Autodesk Fusion 360 part; units mm, degrees
(part 2 of 3)
  arc A350 (118.6572, -98.4677) -> (119.1572, -98.9677) centre (119.1572, -98.4677) ccw
  arc A351 (132.1572, -98.9677) -> (132.6572, -98.4677) centre (132.1572, -98.4677) ccw
  line L356 (138.2072, -84.9677) -> (151.2072, -84.9677)
  line L357 (138.2072, -98.9677) -> (151.2072, -98.9677)
  line L358 (137.7072, -85.4677) -> (137.7072, -98.4677)
  line L359 (151.7072, -85.4677) -> (151.7072, -98.4677)
  arc A352 (138.2072, -84.9677) -> (137.7072, -85.4677) centre (138.2072, -85.4677) ccw
  arc A353 (151.7072, -85.4677) -> (151.2072, -84.9677) centre (151.2072, -85.4677) ccw
  arc A354 (137.7072, -98.4677) -> (138.2072, -98.9677) centre (138.2072, -98.4677) ccw
  arc A355 (151.2072, -98.9677) -> (151.7072, -98.4677) centre (151.2072, -98.4677) ccw
  line L360 (157.2572, -84.9677) -> (170.2572, -84.9677)
  line L361 (157.2572, -98.9677) -> (170.2572, -98.9677)
  line L362 (156.7572, -85.4677) -> (156.7572, -98.4677)
  line L363 (170.7572, -85.4677) -> (170.7572, -98.4677)
  arc A356 (157.2572, -84.9677) -> (156.7572, -85.4677) centre (157.2572, -85.4677) ccw
  arc A357 (170.7572, -85.4677) -> (170.2572, -84.9677) centre (170.2572, -85.4677) ccw
  arc A358 (156.7572, -98.4677) -> (157.2572, -98.9677) centre (157.2572, -98.4677) ccw
  arc A359 (170.2572, -98.9677) -> (170.7572, -98.4677) centre (170.2572, -98.4677) ccw
  line L364 (176.3072, -84.9677) -> (189.3072, -84.9677)
  line L365 (176.3072, -98.9677) -> (189.3072, -98.9677)
  line L366 (175.8072, -85.4677) -> (175.8072, -98.4677)
  line L367 (189.8072, -85.4677) -> (189.8072, -98.4677)
  arc A360 (176.3072, -84.9677) -> (175.8072, -85.4677) centre (176.3072, -85.4677) ccw
  arc A361 (189.8072, -85.4677) -> (189.3072, -84.9677) centre (189.3072, -85.4677) ccw
  arc A362 (175.8072, -98.4677) -> (176.3072, -98.9677) centre (176.3072, -98.4677) ccw
  arc A363 (189.3072, -98.9677) -> (189.8072, -98.4677) centre (189.3072, -98.4677) ccw
  line L368 (195.3572, -84.9677) -> (208.3572, -84.9677)
  line L369 (195.3572, -98.9677) -> (208.3572, -98.9677)
  line L370 (194.8572, -85.4677) -> (194.8572, -98.4677)
  line L371 (208.8572, -85.4677) -> (208.8572, -98.4677)
  arc A364 (195.3572, -84.9677) -> (194.8572, -85.4677) centre (195.3572, -85.4677) ccw
  arc A365 (208.8572, -85.4677) -> (208.3572, -84.9677) centre (208.3572, -85.4677) ccw
  arc A366 (194.8572, -98.4677) -> (195.3572, -98.9677) centre (195.3572, -98.4677) ccw
  arc A367 (208.3572, -98.9677) -> (208.8572, -98.4677) centre (208.3572, -98.4677) ccw
  dimension "d1" = 25.211
  dimension "d2" = 19.875
  constraint horizontal L1
  constraint vertical L0
  constraint horizontal L3
  constraint vertical L2
  measures "d1" distance of L2 L326
  measures "d2" distance of L3 L325
extrude "Extrude1" add sketch "Sketch1" along normal blind 2.5
sketch "Sketch3" plane through (0, 0, 2.5) normal (0, 0, 1) x (-1, 0, 0)
  arc A0 (-66.7697, 65.9177) -> (-66.2697, 66.4177) centre (-66.7697, 66.4177) ccw
  line L0 (-66.7697, 65.9177) -> (-79.7697, 65.9177)
  arc A1 (-80.2697, 66.4177) -> (-79.7697, 65.9177) centre (-79.7697, 66.4177) ccw
  line L1 (-80.2697, 66.4177) -> (-80.2697, 79.4177)
  arc A2 (-79.7697, 79.9177) -> (-80.2697, 79.4177) centre (-79.7697, 79.4177) ccw
  line L2 (-79.7697, 79.9177) -> (-66.7697, 79.9177)
  arc A3 (-66.2697, 79.4177) -> (-66.7697, 79.9177) centre (-66.7697, 79.4177) ccw
  line L3 (-66.2697, 79.4177) -> (-66.2697, 66.4177)
  arc A4 (-195.3572, 8.7677) -> (-194.8572, 9.2677) centre (-195.3572, 9.2677) ccw
  line L4 (-195.3572, 8.7677) -> (-208.3572, 8.7677)
  arc A5 (-208.8572, 9.2677) -> (-208.3572, 8.7677) centre (-208.3572, 9.2677) ccw
  line L5 (-208.8572, 9.2677) -> (-208.8572, 22.2677)
  arc A6 (-208.3572, 22.7677) -> (-208.8572, 22.2677) centre (-208.3572, 22.2677) ccw
  line L6 (-208.3572, 22.7677) -> (-195.3572, 22.7677)
  arc A7 (-194.8572, 22.2677) -> (-195.3572, 22.7677) centre (-195.3572, 22.2677) ccw
  line L7 (-194.8572, 22.2677) -> (-194.8572, 9.2677)
  arc A8 (-14.3822, 27.8177) -> (-13.8822, 28.3177) centre (-14.3822, 28.3177) ccw
  line L8 (-14.3822, 27.8177) -> (-27.3822, 27.8177)
  arc A9 (-27.8822, 28.3177) -> (-27.3822, 27.8177) centre (-27.3822, 28.3177) ccw
  line L9 (-27.8822, 28.3177) -> (-27.8822, 41.3177)
  arc A10 (-27.3822, 41.8177) -> (-27.8822, 41.3177) centre (-27.3822, 41.3177) ccw
  line L10 (-27.3822, 41.8177) -> (-14.3822, 41.8177)
  arc A11 (-13.8822, 41.3177) -> (-14.3822, 41.8177) centre (-14.3822, 41.3177) ccw
  line L11 (-13.8822, 41.3177) -> (-13.8822, 28.3177)
  arc A12 (85.6303, 27.8177) -> (86.1303, 28.3177) centre (85.6303, 28.3177) ccw
  line L12 (85.6303, 27.8177) -> (72.6303, 27.8177)
  arc A13 (72.1303, 28.3177) -> (72.6303, 27.8177) centre (72.6303, 28.3177) ccw
  line L13 (72.1303, 28.3177) -> (72.1303, 41.3177)
  arc A14 (72.6303, 41.8177) -> (72.1303, 41.3177) centre (72.6303, 41.3177) ccw
  line L14 (72.6303, 41.8177) -> (85.6303, 41.8177)
  arc A15 (86.1303, 41.3177) -> (85.6303, 41.8177) centre (85.6303, 41.3177) ccw
  line L15 (86.1303, 41.3177) -> (86.1303, 28.3177)
  arc A16 (-119.1572, -10.2823) -> (-118.6572, -9.7823) centre (-119.1572, -9.7823) ccw
  line L16 (-119.1572, -10.2823) -> (-132.1572, -10.2823)
  arc A17 (-132.6572, -9.7823) -> (-132.1572, -10.2823) centre (-132.1572, -9.7823) ccw
  line L17 (-132.6572, -9.7823) -> (-132.6572, 3.2177)
  arc A18 (-132.1572, 3.7177) -> (-132.6572, 3.2177) centre (-132.1572, 3.2177) ccw
  line L18 (-132.1572, 3.7177) -> (-119.1572, 3.7177)
  arc A19 (-118.6572, 3.2177) -> (-119.1572, 3.7177) centre (-119.1572, 3.2177) ccw
  line L19 (-118.6572, 3.2177) -> (-118.6572, -9.7823)
  arc A20 (-4.8572, -10.2823) -> (-4.3572, -9.7823) centre (-4.8572, -9.7823) ccw
  line L20 (-4.8572, -10.2823) -> (-17.8572, -10.2823)
  arc A21 (-18.3572, -9.7823) -> (-17.8572, -10.2823) centre (-17.8572, -9.7823) ccw
  line L21 (-18.3572, -9.7823) -> (-18.3572, 3.2177)
  arc A22 (-17.8572, 3.7177) -> (-18.3572, 3.2177) centre (-17.8572, 3.2177) ccw
  line L22 (-17.8572, 3.7177) -> (-4.8572, 3.7177)
  arc A23 (-4.3572, 3.2177) -> (-4.8572, 3.7177) centre (-4.8572, 3.2177) ccw
  line L23 (-4.3572, 3.2177) -> (-4.3572, -9.7823)
  arc A24 (-104.8697, 65.9177) -> (-104.3697, 66.4177) centre (-104.8697, 66.4177) ccw
  line L24 (-104.8697, 65.9177) -> (-117.8697, 65.9177)
  arc A25 (-118.3697, 66.4177) -> (-117.8697, 65.9177) centre (-117.8697, 66.4177) ccw
  line L25 (-118.3697, 66.4177) -> (-118.3697, 79.4177)
  arc A26 (-117.8697, 79.9177) -> (-118.3697, 79.4177) centre (-117.8697, 79.4177) ccw
  line L26 (-117.8697, 79.9177) -> (-104.8697, 79.9177)
  arc A27 (-104.3697, 79.4177) -> (-104.8697, 79.9177) centre (-104.8697, 79.4177) ccw
  line L27 (-104.3697, 79.4177) -> (-104.3697, 66.4177)
  arc A28 (-23.9072, -10.2823) -> (-23.4072, -9.7823) centre (-23.9072, -9.7823) ccw
  line L28 (-23.9072, -10.2823) -> (-36.9072, -10.2823)
  arc A29 (-37.4072, -9.7823) -> (-36.9072, -10.2823) centre (-36.9072, -9.7823) ccw
  line L29 (-37.4072, -9.7823) -> (-37.4072, 3.2177)
  arc A30 (-36.9072, 3.7177) -> (-37.4072, 3.2177) centre (-36.9072, 3.2177) ccw
  line L30 (-36.9072, 3.7177) -> (-23.9072, 3.7177)
  arc A31 (-23.4072, 3.2177) -> (-23.9072, 3.7177) centre (-23.9072, 3.2177) ccw
  line L31 (-23.4072, 3.2177) -> (-23.4072, -9.7823)
  arc A32 (52.2928, 8.7677) -> (52.7928, 9.2677) centre (52.2928, 9.2677) ccw
  line L32 (52.2928, 8.7677) -> (39.2928, 8.7677)
  arc A33 (38.7928, 9.2677) -> (39.2928, 8.7677) centre (39.2928, 9.2677) ccw
  line L33 (38.7928, 9.2677) -> (38.7928, 22.2677)
  arc A34 (39.2928, 22.7677) -> (38.7928, 22.2677) centre (39.2928, 22.2677) ccw
  line L34 (39.2928, 22.7677) -> (52.2928, 22.7677)
  arc A35 (52.7928, 22.2677) -> (52.2928, 22.7677) centre (52.2928, 22.2677) ccw
  line L35 (52.7928, 22.2677) -> (52.7928, 9.2677)
  arc A36 (86.9246, 66.9177) -> (87.4246, 67.4177) centre (86.9246, 67.4177) ccw
  line L36 (86.9246, 66.9177) -> (80.9246, 66.9177)
  arc A37 (80.4246, 67.4177) -> (80.9246, 66.9177) centre (80.9246, 67.4177) ccw
  line L37 (80.4246, 67.4177) -> (80.4246, 81.4177)
  arc A38 (80.9246, 81.9177) -> (80.4246, 81.4177) centre (80.9246, 81.4177) ccw
  line L38 (80.9246, 81.9177) -> (86.9246, 81.9177)
  arc A39 (87.4246, 81.4177) -> (86.9246, 81.9177) centre (86.9246, 81.4177) ccw
  line L39 (87.4246, 81.4177) -> (87.4246, 67.4177)
  arc A40 (-155.9629, 47.8677) -> (-155.4629, 48.3677) centre (-155.9629, 48.3677) ccw
  line L40 (-155.9629, 47.8677) -> (-161.9629, 47.8677)
  arc A41 (-162.4629, 48.3677) -> (-161.9629, 47.8677) centre (-161.9629, 48.3677) ccw
  line L41 (-162.4629, 48.3677) -> (-162.4629, 62.3677)
  arc A42 (-161.9629, 62.8677) -> (-162.4629, 62.3677) centre (-161.9629, 62.3677) ccw
  line L42 (-161.9629, 62.8677) -> (-155.9629, 62.8677)
  arc A43 (-155.4629, 62.3677) -> (-155.9629, 62.8677) centre (-155.9629, 62.3677) ccw
  line L43 (-155.4629, 62.3677) -> (-155.4629, 48.3677)
  arc A44 (-23.9072, 8.7677) -> (-23.4072, 9.2677) centre (-23.9072, 9.2677) ccw
  line L44 (-23.9072, 8.7677) -> (-36.9072, 8.7677)
  arc A45 (-37.4072, 9.2677) -> (-36.9072, 8.7677) centre (-36.9072, 9.2677) ccw
  line L45 (-37.4072, 9.2677) -> (-37.4072, 22.2677)
  arc A46 (-36.9072, 22.7677) -> (-37.4072, 22.2677) centre (-36.9072, 22.2677) ccw
  line L46 (-36.9072, 22.7677) -> (-23.9072, 22.7677)
  arc A47 (-23.4072, 22.2677) -> (-23.9072, 22.7677) centre (-23.9072, 22.2677) ccw
  line L47 (-23.4072, 22.2677) -> (-23.4072, 9.2677)
  arc A48 (88.0116, 84.9677) -> (88.5116, 85.4677) centre (88.0116, 85.4677) ccw
  line L48 (88.0116, 84.9677) -> (75.0116, 84.9677)
  arc A49 (74.5116, 85.4677) -> (75.0116, 84.9677) centre (75.0116, 85.4677) ccw
  line L49 (74.5116, 85.4677) -> (74.5116, 98.4677)
  arc A50 (75.0116, 98.9677) -> (74.5116, 98.4677) centre (75.0116, 98.4677) ccw
  line L50 (75.0116, 98.9677) -> (88.0116, 98.9677)
  arc A51 (88.5116, 98.4677) -> (88.0116, 98.9677) centre (88.0116, 98.4677) ccw
  line L51 (88.5116, 98.4677) -> (88.5116, 85.4677)
  arc A52 (-133.4447, 46.8677) -> (-132.9447, 47.3677) centre (-133.4447, 47.3677) ccw
  line L52 (-133.4447, 46.8677) -> (-146.4447, 46.8677)
  arc A53 (-146.9447, 47.3677) -> (-146.4447, 46.8677) centre (-146.4447, 47.3677) ccw
  line L53 (-146.9447, 47.3677) -> (-146.9447, 60.3677)
  arc A54 (-146.4447, 60.8677) -> (-146.9447, 60.3677) centre (-146.4447, 60.3677) ccw
  line L54 (-146.4447, 60.8677) -> (-133.4447, 60.8677)
  arc A55 (-132.9447, 60.3677) -> (-133.4447, 60.8677) centre (-133.4447, 60.3677) ccw
  line L55 (-132.9447, 60.3677) -> (-132.9447, 47.3677)
  arc A56 (-171.5447, 27.8177) -> (-171.0447, 28.3177) centre (-171.5447, 28.3177) ccw
  line L56 (-171.5447, 27.8177) -> (-184.5447, 27.8177)
  arc A57 (-185.0447, 28.3177) -> (-184.5447, 27.8177) centre (-184.5447, 28.3177) ccw
  line L57 (-185.0447, 28.3177) -> (-185.0447, 41.3177)
  arc A58 (-184.5447, 41.8177) -> (-185.0447, 41.3177) centre (-184.5447, 41.3177) ccw
  line L58 (-184.5447, 41.8177) -> (-171.5447, 41.8177)
  arc A59 (-171.0447, 41.3177) -> (-171.5447, 41.8177) centre (-171.5447, 41.3177) ccw
  line L59 (-171.0447, 41.3177) -> (-171.0447, 28.3177)
  arc A60 (-138.2072, -10.2823) -> (-137.7072, -9.7823) centre (-138.2072, -9.7823) ccw
  line L60 (-138.2072, -10.2823) -> (-151.2072, -10.2823)
  arc A61 (-151.7072, -9.7823) -> (-151.2072, -10.2823) centre (-151.2072, -9.7823) ccw
  line L61 (-151.7072, -9.7823) -> (-151.7072, 3.2177)
  arc A62 (-151.2072, 3.7177) -> (-151.7072, 3.2177) centre (-151.2072, 3.2177) ccw
  line L62 (-151.2072, 3.7177) -> (-138.2072, 3.7177)
  arc A63 (-137.7072, 3.2177) -> (-138.2072, 3.7177) centre (-138.2072, 3.2177) ccw
  line L63 (-137.7072, 3.2177) -> (-137.7072, -9.7823)
  arc A64 (-176.3072, -10.2823) -> (-175.8072, -9.7823) centre (-176.3072, -9.7823) ccw
  line L64 (-176.3072, -10.2823) -> (-189.3072, -10.2823)
  arc A65 (-189.8072, -9.7823) -> (-189.3072, -10.2823) centre (-189.3072, -9.7823) ccw
  line L65 (-189.8072, -9.7823) -> (-189.8072, 3.2177)
  arc A66 (-189.3072, 3.7177) -> (-189.8072, 3.2177) centre (-189.3072, 3.2177) ccw
  line L66 (-189.3072, 3.7177) -> (-176.3072, 3.7177)
  arc A67 (-175.8072, 3.2177) -> (-176.3072, 3.7177) centre (-176.3072, 3.2177) ccw
  line L67 (-175.8072, 3.2177) -> (-175.8072, -9.7823)
  arc A68 (4.6678, 27.8177) -> (5.1678, 28.3177) centre (4.6678, 28.3177) ccw
  line L68 (4.6678, 27.8177) -> (-8.3322, 27.8177)
  arc A69 (-8.8322, 28.3177) -> (-8.3322, 27.8177) centre (-8.3322, 28.3177) ccw
  line L69 (-8.8322, 28.3177) -> (-8.8322, 41.3177)
  arc A70 (-8.3322, 41.8177) -> (-8.8322, 41.3177) centre (-8.3322, 41.3177) ccw
  line L70 (-8.3322, 41.8177) -> (4.6678, 41.8177)
  arc A71 (5.1678, 41.3177) -> (4.6678, 41.8177) centre (4.6678, 41.3177) ccw
  line L71 (5.1678, 41.3177) -> (5.1678, 28.3177)
  arc A72 (64.1991, 84.9677) -> (64.6991, 85.4677) centre (64.1991, 85.4677) ccw
  line L72 (64.1991, 84.9677) -> (51.1991, 84.9677)
  arc A73 (50.6991, 85.4677) -> (51.1991, 84.9677) centre (51.1991, 85.4677) ccw
  line L73 (50.6991, 85.4677) -> (50.6991, 98.4677)
  arc A74 (51.1991, 98.9677) -> (50.6991, 98.4677) centre (51.1991, 98.4677) ccw
  line L74 (51.1991, 98.9677) -> (64.1991, 98.9677)
  arc A75 (64.6991, 98.4677) -> (64.1991, 98.9677) centre (64.1991, 98.4677) ccw
  line L75 (64.6991, 98.4677) -> (64.6991, 85.4677)
  arc A76 (52.2928, -10.2823) -> (52.7928, -9.7823) centre (52.2928, -9.7823) ccw
  line L76 (52.2928, -10.2823) -> (39.2928, -10.2823)
  arc A77 (38.7928, -9.7823) -> (39.2928, -10.2823) centre (39.2928, -9.7823) ccw
  line L77 (38.7928, -9.7823) -> (38.7928, 3.2177)
  arc A78 (39.2928, 3.7177) -> (38.7928, 3.2177) centre (39.2928, 3.2177) ccw
  line L78 (39.2928, 3.7177) -> (52.2928, 3.7177)
  arc A79 (52.7928, 3.2177) -> (52.2928, 3.7177) centre (52.2928, 3.2177) ccw
  line L79 (52.7928, 3.2177) -> (52.7928, -9.7823)
  arc A80 (-109.6322, 27.8177) -> (-109.1322, 28.3177) centre (-109.6322, 28.3177) ccw
  line L80 (-109.6322, 27.8177) -> (-122.6322, 27.8177)
  arc A81 (-123.1322, 28.3177) -> (-122.6322, 27.8177) centre (-122.6322, 28.3177) ccw
  line L81 (-123.1322, 28.3177) -> (-123.1322, 41.3177)
  arc A82 (-122.6322, 41.8177) -> (-123.1322, 41.3177) centre (-122.6322, 41.3177) ccw
  line L82 (-122.6322, 41.8177) -> (-109.6322, 41.8177)
  arc A83 (-109.1322, 41.3177) -> (-109.6322, 41.8177) centre (-109.6322, 41.3177) ccw
  line L83 (-109.1322, 41.3177) -> (-109.1322, 28.3177)
  arc A84 (42.7678, 27.8177) -> (43.2678, 28.3177) centre (42.7678, 28.3177) ccw
  line L84 (42.7678, 27.8177) -> (29.7678, 27.8177)
  arc A85 (29.2678, 28.3177) -> (29.7678, 27.8177) centre (29.7678, 28.3177) ccw
  line L85 (29.2678, 28.3177) -> (29.2678, 41.3177)
  arc A86 (29.7678, 41.8177) -> (29.2678, 41.3177) centre (29.7678, 41.3177) ccw
  line L86 (29.7678, 41.8177) -> (42.7678, 41.8177)
  arc A87 (43.2678, 41.3177) -> (42.7678, 41.8177) centre (42.7678, 41.3177) ccw
  line L87 (43.2678, 41.3177) -> (43.2678, 28.3177)
  arc A88 (-100.1072, 8.7677) -> (-99.6072, 9.2677) centre (-100.1072, 9.2677) ccw
  line L88 (-100.1072, 8.7677) -> (-113.1072, 8.7677)
  arc A89 (-113.6072, 9.2677) -> (-113.1072, 8.7677) centre (-113.1072, 9.2677) ccw
  line L89 (-113.6072, 9.2677) -> (-113.6072, 22.2677)
  arc A90 (-113.1072, 22.7677) -> (-113.6072, 22.2677) centre (-113.1072, 22.2677) ccw
  line L90 (-113.1072, 22.7677) -> (-100.1072, 22.7677)
  arc A91 (-99.6072, 22.2677) -> (-100.1072, 22.7677) centre (-100.1072, 22.2677) ccw
  line L91 (-99.6072, 22.2677) -> (-99.6072, 9.2677)
  arc A92 (-0.0947, 46.8677) -> (0.4053, 47.3677) centre (-0.0947, 47.3677) ccw
  line L92 (-0.0947, 46.8677) -> (-13.0947, 46.8677)
  arc A93 (-13.5947, 47.3677) -> (-13.0947, 46.8677) centre (-13.0947, 47.3677) ccw
  line L93 (-13.5947, 47.3677) -> (-13.5947, 60.3677)
  arc A94 (-13.0947, 60.8677) -> (-13.5947, 60.3677) centre (-13.0947, 60.3677) ccw
  line L94 (-13.0947, 60.8677) -> (-0.0947, 60.8677)
  arc A95 (0.4053, 60.3677) -> (-0.0947, 60.8677) centre (-0.0947, 60.3677) ccw
  line L95 (0.4053, 60.3677) -> (0.4053, 47.3677)
  arc A96 (63.0486, 66.9177) -> (63.5486, 67.4177) centre (63.0486, 67.4177) ccw
  line L96 (63.0486, 66.9177) -> (57.0486, 66.9177)
  arc A97 (56.5486, 67.4177) -> (57.0486, 66.9177) centre (57.0486, 67.4177) ccw
  line L97 (56.5486, 67.4177) -> (56.5486, 81.4177)
  arc A98 (57.0486, 81.9177) -> (56.5486, 81.4177) centre (57.0486, 81.4177) ccw
  line L98 (57.0486, 81.9177) -> (63.0486, 81.9177)
  arc A99 (63.5486, 81.4177) -> (63.0486, 81.9177) centre (63.0486, 81.4177) ccw
  line L99 (63.5486, 81.4177) -> (63.5486, 67.4177)
  arc A100 (-33.4322, 27.8177) -> (-32.9322, 28.3177) centre (-33.4322, 28.3177) ccw
  line L100 (-33.4322, 27.8177) -> (-46.4322, 27.8177)
  arc A101 (-46.9322, 28.3177) -> (-46.4322, 27.8177) centre (-46.4322, 28.3177) ccw
  line L101 (-46.9322, 28.3177) -> (-46.9322, 41.3177)
  arc A102 (-46.4322, 41.8177) -> (-46.9322, 41.3177) centre (-46.4322, 41.3177) ccw
  line L102 (-46.4322, 41.8177) -> (-33.4322, 41.8177)
  arc A103 (-32.9322, 41.3177) -> (-33.4322, 41.8177) centre (-33.4322, 41.3177) ccw
  line L103 (-32.9322, 41.3177) -> (-32.9322, 28.3177)
  arc A104 (-195.3572, 27.8177) -> (-194.8572, 28.3177) centre (-195.3572, 28.3177) ccw
  line L104 (-195.3572, 27.8177) -> (-208.3572, 27.8177)
  arc A105 (-208.8572, 28.3177) -> (-208.3572, 27.8177) centre (-208.3572, 28.3177) ccw
  line L105 (-208.8572, 28.3177) -> (-208.8572, 41.3177)
  arc A106 (-208.3572, 41.8177) -> (-208.8572, 41.3177) centre (-208.3572, 41.3177) ccw
  line L106 (-208.3572, 41.8177) -> (-195.3572, 41.8177)
  arc A107 (-194.8572, 41.3177) -> (-195.3572, 41.8177) centre (-195.3572, 41.3177) ccw
  line L107 (-194.8572, 41.3177) -> (-194.8572, 28.3177)
  arc A108 (-176.3072, 65.9177) -> (-175.8072, 66.4177) centre (-176.3072, 66.4177) ccw
  line L108 (-176.3072, 65.9177) -> (-189.3072, 65.9177)
  arc A109 (-189.8072, 66.4177) -> (-189.3072, 65.9177) centre (-189.3072, 66.4177) ccw
  line L109 (-189.8072, 66.4177) -> (-189.8072, 79.4177)
  arc A110 (-189.3072, 79.9177) -> (-189.8072, 79.4177) centre (-189.3072, 79.4177) ccw
  line L110 (-189.3072, 79.9177) -> (-176.3072, 79.9177)
  arc A111 (-175.8072, 79.4177) -> (-176.3072, 79.9177) centre (-176.3072, 79.4177) ccw
  line L111 (-175.8072, 79.4177) -> (-175.8072, 66.4177)
  arc A112 (-100.1072, -10.2823) -> (-99.6072, -9.7823) centre (-100.1072, -9.7823) ccw
  line L112 (-100.1072, -10.2823) -> (-113.1072, -10.2823)
  arc A113 (-113.6072, -9.7823) -> (-113.1072, -10.2823) centre (-113.1072, -9.7823) ccw
  line L113 (-113.6072, -9.7823) -> (-113.6072, 3.2177)
  arc A114 (-113.1072, 3.7177) -> (-113.6072, 3.2177) centre (-113.1072, 3.2177) ccw
  line L114 (-113.1072, 3.7177) -> (-100.1072, 3.7177)
  arc A115 (-99.6072, 3.2177) -> (-100.1072, 3.7177) centre (-100.1072, 3.2177) ccw
  line L115 (-99.6072, 3.2177) -> (-99.6072, -9.7823)
  arc A116 (-157.2572, -10.2823) -> (-156.7572, -9.7823) centre (-157.2572, -9.7823) ccw
  line L116 (-157.2572, -10.2823) -> (-170.2572, -10.2823)
  arc A117 (-170.7572, -9.7823) -> (-170.2572, -10.2823) centre (-170.2572, -9.7823) ccw
  line L117 (-170.7572, -9.7823) -> (-170.7572, 3.2177)
  arc A118 (-170.2572, 3.7177) -> (-170.7572, 3.2177) centre (-170.2572, 3.2177) ccw
  line L118 (-170.2572, 3.7177) -> (-157.2572, 3.7177)
  arc A119 (-156.7572, 3.2177) -> (-157.2572, 3.7177) centre (-157.2572, 3.2177) ccw
  line L119 (-156.7572, 3.2177) -> (-156.7572, -9.7823)
  arc A120 (33.2428, 8.7677) -> (33.7428, 9.2677) centre (33.2428, 9.2677) ccw
  line L120 (33.2428, 8.7677) -> (20.2428, 8.7677)
  arc A121 (19.7428, 9.2677) -> (20.2428, 8.7677) centre (20.2428, 9.2677) ccw
  line L121 (19.7428, 9.2677) -> (19.7428, 22.2677)
  arc A122 (20.2428, 22.7677) -> (19.7428, 22.2677) centre (20.2428, 22.2677) ccw
  line L122 (20.2428, 22.7677) -> (33.2428, 22.7677)
  arc A123 (33.7428, 22.2677) -> (33.2428, 22.7677) centre (33.2428, 22.2677) ccw
  line L123 (33.7428, 22.2677) -> (33.7428, 9.2677)
  arc A124 (90.3928, -10.2823) -> (90.8928, -9.7823) centre (90.3928, -9.7823) ccw
  line L124 (90.3928, -10.2823) -> (77.3928, -10.2823)
  arc A125 (76.8928, -9.7823) -> (77.3928, -10.2823) centre (77.3928, -9.7823) ccw
  line L125 (76.8928, -9.7823) -> (76.8928, 3.2177)
  arc A126 (77.3928, 3.7177) -> (76.8928, 3.2177) centre (77.3928, 3.2177) ccw
  line L126 (77.3928, 3.7177) -> (90.3928, 3.7177)
  arc A127 (90.8928, 3.2177) -> (90.3928, 3.7177) centre (90.3928, 3.2177) ccw
  line L127 (90.8928, 3.2177) -> (90.8928, -9.7823)
  arc A128 (18.9553, 46.8677) -> (19.4553, 47.3677) centre (18.9553, 47.3677) ccw
  line L128 (18.9553, 46.8677) -> (5.9553, 46.8677)
  arc A129 (5.4553, 47.3677) -> (5.9553, 46.8677) centre (5.9553, 47.3677) ccw
  line L129 (5.4553, 47.3677) -> (5.4553, 60.3677)
  arc A130 (5.9553, 60.8677) -> (5.4553, 60.3677) centre (5.9553, 60.3677) ccw
  line L130 (5.9553, 60.8677) -> (18.9553, 60.8677)
  arc A131 (19.4553, 60.3677) -> (18.9553, 60.8677) centre (18.9553, 60.3677) ccw
  line L131 (19.4553, 60.3677) -> (19.4553, 47.3677)
  arc A132 (-71.5322, 27.8177) -> (-71.0322, 28.3177) centre (-71.5322, 28.3177) ccw
  line L132 (-71.5322, 27.8177) -> (-84.5322, 27.8177)
  arc A133 (-85.0322, 28.3177) -> (-84.5322, 27.8177) centre (-84.5322, 28.3177) ccw
  line L133 (-85.0322, 28.3177) -> (-85.0322, 41.3177)
  arc A134 (-84.5322, 41.8177) -> (-85.0322, 41.3177) centre (-84.5322, 41.3177) ccw
  line L134 (-84.5322, 41.8177) -> (-71.5322, 41.8177)
  arc A135 (-71.0322, 41.3177) -> (-71.5322, 41.8177) centre (-71.5322, 41.3177) ccw
  line L135 (-71.0322, 41.3177) -> (-71.0322, 28.3177)
  arc A136 (-114.3947, 46.8677) -> (-113.8947, 47.3677) centre (-114.3947, 47.3677) ccw
  line L136 (-114.3947, 46.8677) -> (-127.3947, 46.8677)
  arc A137 (-127.8947, 47.3677) -> (-127.3947, 46.8677) centre (-127.3947, 47.3677) ccw
  line L137 (-127.8947, 47.3677) -> (-127.8947, 60.3677)
  arc A138 (-127.3947, 60.8677) -> (-127.8947, 60.3677) centre (-127.3947, 60.3677) ccw
  line L138 (-127.3947, 60.8677) -> (-114.3947, 60.8677)
  arc A139 (-113.8947, 60.3677) -> (-114.3947, 60.8677) centre (-114.3947, 60.3677) ccw
  line L139 (-113.8947, 60.3677) -> (-113.8947, 47.3677)
  arc A140 (-81.0572, -10.2823) -> (-80.5572, -9.7823) centre (-81.0572, -9.7823) ccw
  line L140 (-81.0572, -10.2823) -> (-94.0572, -10.2823)
  arc A141 (-94.5572, -9.7823) -> (-94.0572, -10.2823) centre (-94.0572, -9.7823) ccw
  line L141 (-94.5572, -9.7823) -> (-94.5572, 3.2177)
  arc A142 (-94.0572, 3.7177) -> (-94.5572, 3.2177) centre (-94.0572, 3.2177) ccw
  line L142 (-94.0572, 3.7177) -> (-81.0572, 3.7177)
  arc A143 (-80.5572, 3.2177) -> (-81.0572, 3.7177) centre (-81.0572, 3.2177) ccw
  line L143 (-80.5572, 3.2177) -> (-80.5572, -9.7823)
  arc A144 (15.4491, 85.9677) -> (15.9491, 86.4677) centre (15.4491, 86.4677) ccw
  line L144 (15.4491, 85.9677) -> (9.4491, 85.9677)
  arc A145 (8.9491, 86.4677) -> (9.4491, 85.9677) centre (9.4491, 86.4677) ccw
  line L145 (8.9491, 86.4677) -> (8.9491, 100.4677)
  arc A146 (9.4491, 100.9677) -> (8.9491, 100.4677) centre (9.4491, 100.4677) ccw
  line L146 (9.4491, 100.9677) -> (15.4491, 100.9677)
  arc A147 (15.9491, 100.4677) -> (15.4491, 100.9677) centre (15.4491, 100.4677) ccw
  line L147 (15.9491, 100.4677) -> (15.9491, 86.4677)
  arc A148 (-195.3572, 84.9677) -> (-194.8572, 85.4677) centre (-195.3572, 85.4677) ccw
  line L148 (-195.3572, 84.9677) -> (-208.3572, 84.9677)
  arc A149 (-208.8572, 85.4677) -> (-208.3572, 84.9677) centre (-208.3572, 85.4677) ccw
  line L149 (-208.8572, 85.4677) -> (-208.8572, 98.4677)
  arc A150 (-208.3572, 98.9677) -> (-208.8572, 98.4677) centre (-208.3572, 98.4677) ccw
  line L150 (-208.3572, 98.9677) -> (-195.3572, 98.9677)
  arc A151 (-194.8572, 98.4677) -> (-195.3572, 98.9677) centre (-195.3572, 98.4677) ccw
  line L151 (-194.8572, 98.4677) -> (-194.8572, 85.4677)
  arc A152 (-138.2072, 84.9677) -> (-137.7072, 85.4677) centre (-138.2072, 85.4677) ccw
  line L152 (-138.2072, 84.9677) -> (-151.2072, 84.9677)
  arc A153 (-151.7072, 85.4677) -> (-151.2072, 84.9677) centre (-151.2072, 85.4677) ccw
  line L153 (-151.7072, 85.4677) -> (-151.7072, 98.4677)
  arc A154 (-151.2072, 98.9677) -> (-151.7072, 98.4677) centre (-151.2072, 98.4677) ccw
  line L154 (-151.2072, 98.9677) -> (-138.2072, 98.9677)
  arc A155 (-137.7072, 98.4677) -> (-138.2072, 98.9677) centre (-138.2072, 98.4677) ccw
  line L155 (-137.7072, 98.4677) -> (-137.7072, 85.4677)
  arc A156 (83.2491, 46.8677) -> (83.7491, 47.3677) centre (83.2491, 47.3677) ccw
  line L156 (83.2491, 46.8677) -> (70.2491, 46.8677)
  arc A157 (69.7491, 47.3677) -> (70.2491, 46.8677) centre (70.2491, 47.3677) ccw
  line L157 (69.7491, 47.3677) -> (69.7491, 60.3677)
  arc A158 (70.2491, 60.8677) -> (69.7491, 60.3677) centre (70.2491, 60.3677) ccw
  line L158 (70.2491, 60.8677) -> (83.2491, 60.8677)
  arc A159 (83.7491, 60.3677) -> (83.2491, 60.8677) centre (83.2491, 60.3677) ccw
  line L159 (83.7491, 60.3677) -> (83.7491, 47.3677)
  arc A160 (-166.7822, 8.7677) -> (-166.2822, 9.2677) centre (-166.7822, 9.2677) ccw
  line L160 (-166.7822, 8.7677) -> (-179.7822, 8.7677)
  arc A161 (-180.2822, 9.2677) -> (-179.7822, 8.7677) centre (-179.7822, 9.2677) ccw
  line L161 (-180.2822, 9.2677) -> (-180.2822, 22.2677)
  arc A162 (-179.7822, 22.7677) -> (-180.2822, 22.2677) centre (-179.7822, 22.2677) ccw
  line L162 (-179.7822, 22.7677) -> (-166.7822, 22.7677)
  arc A163 (-166.2822, 22.2677) -> (-166.7822, 22.7677) centre (-166.7822, 22.2677) ccw
  line L163 (-166.2822, 22.2677) -> (-166.2822, 9.2677)
  arc A164 (-195.3572, 46.8677) -> (-194.8572, 47.3677) centre (-195.3572, 47.3677) ccw
  line L164 (-195.3572, 46.8677) -> (-208.3572, 46.8677)
  arc A165 (-208.8572, 47.3677) -> (-208.3572, 46.8677) centre (-208.3572, 47.3677) ccw
  line L165 (-208.8572, 47.3677) -> (-208.8572, 60.3677)
  arc A166 (-208.3572, 60.8677) -> (-208.8572, 60.3677) centre (-208.3572, 60.3677) ccw
  line L166 (-208.3572, 60.8677) -> (-195.3572, 60.8677)
  arc A167 (-194.8572, 60.3677) -> (-195.3572, 60.8677) centre (-195.3572, 60.3677) ccw
  line L167 (-194.8572, 60.3677) -> (-194.8572, 47.3677)
  line L168 (-228.9474, 118.8427) -> (-228.9474, -57.4273)
  line L169 (-228.9474, -57.4273) -> (113.7226, -57.4273)
  line L170 (113.7226, -57.4273) -> (113.7226, 118.8427)
  line L171 (113.7226, 118.8427) -> (-228.9474, 118.8427)
  arc A168 (-182.2202, 9.7677) -> (-181.7202, 10.2677) centre (-182.2202, 10.2677) ccw
  line L172 (-182.2202, 9.7677) -> (-188.2202, 9.7677)
  arc A169 (-188.7202, 10.2677) -> (-188.2202, 9.7677) centre (-188.2202, 10.2677) ccw
  line L173 (-188.7202, 10.2677) -> (-188.7202, 24.2677)
  arc A170 (-188.2202, 24.7677) -> (-188.7202, 24.2677) centre (-188.2202, 24.2677) ccw
  line L174 (-188.2202, 24.7677) -> (-182.2202, 24.7677)
  arc A171 (-181.7202, 24.2677) -> (-182.2202, 24.7677) centre (-182.2202, 24.2677) ccw
  line L175 (-181.7202, 24.2677) -> (-181.7202, 10.2677)
  arc A172 (-76.2947, 46.8677) -> (-75.7947, 47.3677) centre (-76.2947, 47.3677) ccw
  line L176 (-76.2947, 46.8677) -> (-89.2947, 46.8677)
  arc A173 (-89.7947, 47.3677) -> (-89.2947, 46.8677) centre (-89.2947, 47.3677) ccw
  line L177 (-89.7947, 47.3677) -> (-89.7947, 60.3677)
  arc A174 (-89.2947, 60.8677) -> (-89.7947, 60.3677) centre (-89.2947, 60.3677) ccw
  line L178 (-89.2947, 60.8677) -> (-76.2947, 60.8677)
  arc A175 (-75.7947, 60.3677) -> (-76.2947, 60.8677) centre (-76.2947, 60.3677) ccw
  line L179 (-75.7947, 60.3677) -> (-75.7947, 47.3677)
  arc A176 (-138.2072, 8.7677) -> (-137.7072, 9.2677) centre (-138.2072, 9.2677) ccw
  line L180 (-138.2072, 8.7677) -> (-151.2072, 8.7677)
  arc A177 (-151.7072, 9.2677) -> (-151.2072, 8.7677) centre (-151.2072, 9.2677) ccw
  line L181 (-151.7072, 9.2677) -> (-151.7072, 22.2677)
  arc A178 (-151.2072, 22.7677) -> (-151.7072, 22.2677) centre (-151.2072, 22.2677) ccw
  line L182 (-151.2072, 22.7677) -> (-138.2072, 22.7677)
  arc A179 (-137.7072, 22.2677) -> (-138.2072, 22.7677) centre (-138.2072, 22.2677) ccw
  line L183 (-137.7072, 22.2677) -> (-137.7072, 9.2677)
  arc A180 (-164.4009, 46.8677) -> (-163.9009, 47.3677) centre (-164.4009, 47.3677) ccw
  line L184 (-164.4009, 46.8677) -> (-177.4009, 46.8677)
  arc A181 (-177.9009, 47.3677) -> (-177.4009, 46.8677) centre (-177.4009, 47.3677) ccw
  line L185 (-177.9009, 47.3677) -> (-177.9009, 60.3677)
  arc A182 (-177.4009, 60.8677) -> (-177.9009, 60.3677) centre (-177.4009, 60.3677) ccw
  line L186 (-177.4009, 60.8677) -> (-164.4009, 60.8677)
  arc A183 (-163.9009, 60.3677) -> (-164.4009, 60.8677) centre (-164.4009, 60.3677) ccw
  line L187 (-163.9009, 60.3677) -> (-163.9009, 47.3677)
  arc A184 (-42.9572, 8.7677) -> (-42.4572, 9.2677) centre (-42.9572, 9.2677) ccw
  line L188 (-42.9572, 8.7677) -> (-55.9572, 8.7677)
  arc A185 (-56.4572, 9.2677) -> (-55.9572, 8.7677) centre (-55.9572, 9.2677) ccw
  line L189 (-56.4572, 9.2677) -> (-56.4572, 22.2677)
  arc A186 (-55.9572, 22.7677) -> (-56.4572, 22.2677) centre (-55.9572, 22.2677) ccw
  line L190 (-55.9572, 22.7677) -> (-42.9572, 22.7677)
  arc A187 (-42.4572, 22.2677) -> (-42.9572, 22.7677) centre (-42.9572, 22.2677) ccw
  line L191 (-42.4572, 22.2677) -> (-42.4572, 9.2677)
  arc A188 (-128.6822, 27.8177) -> (-128.1822, 28.3177) centre (-128.6822, 28.3177) ccw
  line L192 (-128.6822, 27.8177) -> (-141.6822, 27.8177)
  arc A189 (-142.1822, 28.3177) -> (-141.6822, 27.8177) centre (-141.6822, 28.3177) ccw
  line L193 (-142.1822, 28.3177) -> (-142.1822, 41.3177)
  arc A190 (-141.6822, 41.8177) -> (-142.1822, 41.3177) centre (-141.6822, 41.3177) ccw
  line L194 (-141.6822, 41.8177) -> (-128.6822, 41.8177)
  arc A191 (-128.1822, 41.3177) -> (-128.6822, 41.8177) centre (-128.6822, 41.3177) ccw
  line L195 (-128.1822, 41.3177) -> (-128.1822, 28.3177)
  arc A192 (-28.6697, 65.9177) -> (-28.1697, 66.4177) centre (-28.6697, 66.4177) ccw
  line L196 (-28.6697, 65.9177) -> (-41.6697, 65.9177)
  arc A193 (-42.1697, 66.4177) -> (-41.6697, 65.9177) centre (-41.6697, 66.4177) ccw
  line L197 (-42.1697, 66.4177) -> (-42.1697, 79.4177)
  arc A194 (-41.6697, 79.9177) -> (-42.1697, 79.4177) centre (-41.6697, 79.4177) ccw
  line L198 (-41.6697, 79.9177) -> (-28.6697, 79.9177)
  arc A195 (-28.1697, 79.4177) -> (-28.6697, 79.9177) centre (-28.6697, 79.4177) ccw
  line L199 (-28.1697, 79.4177) -> (-28.1697, 66.4177)
  arc A196 (78.4866, 65.9177) -> (78.9866, 66.4177) centre (78.4866, 66.4177) ccw
  line L200 (78.4866, 65.9177) -> (65.4866, 65.9177)
  arc A197 (64.9866, 66.4177) -> (65.4866, 65.9177) centre (65.4866, 66.4177) ccw
  line L201 (64.9866, 66.4177) -> (64.9866, 79.4177)
  arc A198 (65.4866, 79.9177) -> (64.9866, 79.4177) centre (65.4866, 79.4177) ccw
  line L202 (65.4866, 79.9177) -> (78.4866, 79.9177)
  arc A199 (78.9866, 79.4177) -> (78.4866, 79.9177) centre (78.4866, 79.4177) ccw
  line L203 (78.9866, 79.4177) -> (78.9866, 66.4177)
  arc A200 (-100.1072, 84.9677) -> (-99.6072, 85.4677) centre (-100.1072, 85.4677) ccw
  line L204 (-100.1072, 84.9677) -> (-113.1072, 84.9677)
  arc A201 (-113.6072, 85.4677) -> (-113.1072, 84.9677) centre (-113.1072, 85.4677) ccw
  line L205 (-113.6072, 85.4677) -> (-113.6072, 98.4677)
  arc A202 (-113.1072, 98.9677) -> (-113.6072, 98.4677) centre (-113.1072, 98.4677) ccw
  line L206 (-113.1072, 98.9677) -> (-100.1072, 98.9677)
  arc A203 (-99.6072, 98.4677) -> (-100.1072, 98.9677) centre (-100.1072, 98.4677) ccw
  line L207 (-99.6072, 98.4677) -> (-99.6072, 85.4677)
  arc A204 (-119.1572, 84.9677) -> (-118.6572, 85.4677) centre (-119.1572, 85.4677) ccw
  line L208 (-119.1572, 84.9677) -> (-132.1572, 84.9677)
  arc A205 (-132.6572, 85.4677) -> (-132.1572, 84.9677) centre (-132.1572, 85.4677) ccw
  line L209 (-132.6572, 85.4677) -> (-132.6572, 98.4677)
  arc A206 (-132.1572, 98.9677) -> (-132.6572, 98.4677) centre (-132.1572, 98.4677) ccw
  line L210 (-132.1572, 98.9677) -> (-119.1572, 98.9677)
  arc A207 (-118.6572, 98.4677) -> (-119.1572, 98.9677) centre (-119.1572, 98.4677) ccw
  line L211 (-118.6572, 98.4677) -> (-118.6572, 85.4677)
  arc A208 (-119.1572, 8.7677) -> (-118.6572, 9.2677) centre (-119.1572, 9.2677) ccw
  line L212 (-119.1572, 8.7677) -> (-132.1572, 8.7677)
  arc A209 (-132.6572, 9.2677) -> (-132.1572, 8.7677) centre (-132.1572, 9.2677) ccw
  line L213 (-132.6572, 9.2677) -> (-132.6572, 22.2677)
  arc A210 (-132.1572, 22.7677) -> (-132.6572, 22.2677) centre (-132.1572, 22.2677) ccw
  line L214 (-132.1572, 22.7677) -> (-119.1572, 22.7677)
  arc A211 (-118.6572, 22.2677) -> (-119.1572, 22.7677) centre (-119.1572, 22.2677) ccw
  line L215 (-118.6572, 22.2677) -> (-118.6572, 9.2677)
  arc A212 (-157.2572, 84.9677) -> (-156.7572, 85.4677) centre (-157.2572, 85.4677) ccw
  line L216 (-157.2572, 84.9677) -> (-170.2572, 84.9677)
  arc A213 (-170.7572, 85.4677) -> (-170.2572, 84.9677) centre (-170.2572, 85.4677) ccw
  line L217 (-170.7572, 85.4677) -> (-170.7572, 98.4677)
  arc A214 (-170.2572, 98.9677) -> (-170.7572, 98.4677) centre (-170.2572, 98.4677) ccw
  line L218 (-170.2572, 98.9677) -> (-157.2572, 98.9677)
  arc A215 (-156.7572, 98.4677) -> (-157.2572, 98.9677) centre (-157.2572, 98.4677) ccw
  line L219 (-156.7572, 98.4677) -> (-156.7572, 85.4677)
  arc A216 (-57.2447, 46.8677) -> (-56.7447, 47.3677) centre (-57.2447, 47.3677) ccw
  line L220 (-57.2447, 46.8677) -> (-70.2447, 46.8677)
  arc A217 (-70.7447, 47.3677) -> (-70.2447, 46.8677) centre (-70.2447, 47.3677) ccw
  line L221 (-70.7447, 47.3677) -> (-70.7447, 60.3677)
  arc A218 (-70.2447, 60.8677) -> (-70.7447, 60.3677) centre (-70.2447, 60.3677) ccw
  line L222 (-70.2447, 60.8677) -> (-57.2447, 60.8677)
  arc A219 (-56.7447, 60.3677) -> (-57.2447, 60.8677) centre (-57.2447, 60.3677) ccw
  line L223 (-56.7447, 60.3677) -> (-56.7447, 47.3677)
  arc A220 (-42.9572, -10.2823) -> (-42.4572, -9.7823) centre (-42.9572, -9.7823) ccw
  line L224 (-42.9572, -10.2823) -> (-55.9572, -10.2823)
  arc A221 (-56.4572, -9.7823) -> (-55.9572, -10.2823) centre (-55.9572, -9.7823) ccw
  line L225 (-56.4572, -9.7823) -> (-56.4572, 3.2177)
  arc A222 (-55.9572, 3.7177) -> (-56.4572, 3.2177) centre (-55.9572, 3.2177) ccw
  line L226 (-55.9572, 3.7177) -> (-42.9572, 3.7177)
  arc A223 (-42.4572, 3.2177) -> (-42.9572, 3.7177) centre (-42.9572, 3.2177) ccw
  line L227 (-42.4572, 3.2177) -> (-42.4572, -9.7823)
  arc A224 (40.3866, 84.9677) -> (40.8866, 85.4677) centre (40.3866, 85.4677) ccw
  line L228 (40.3866, 84.9677) -> (27.3866, 84.9677)
  arc A225 (26.8866, 85.4677) -> (27.3866, 84.9677) centre (27.3866, 85.4677) ccw
  line L229 (26.8866, 85.4677) -> (26.8866, 98.4677)
  arc A226 (27.3866, 98.9677) -> (26.8866, 98.4677) centre (27.3866, 98.4677) ccw
  line L230 (27.3866, 98.9677) -> (40.3866, 98.9677)
  arc A227 (40.8866, 98.4677) -> (40.3866, 98.9677) centre (40.3866, 98.4677) ccw
  line L231 (40.8866, 98.4677) -> (40.8866, 85.4677)
  arc A228 (-158.3442, 9.7677) -> (-157.8442, 10.2677) centre (-158.3442, 10.2677) ccw
  line L232 (-158.3442, 9.7677) -> (-164.3442, 9.7677)
  arc A229 (-164.8442, 10.2677) -> (-164.3442, 9.7677) centre (-164.3442, 10.2677) ccw
  line L233 (-164.8442, 10.2677) -> (-164.8442, 24.2677)
  arc A230 (-164.3442, 24.7677) -> (-164.8442, 24.2677) centre (-164.3442, 24.2677) ccw
  line L234 (-164.3442, 24.7677) -> (-158.3442, 24.7677)
  arc A231 (-157.8442, 24.2677) -> (-158.3442, 24.7677) centre (-158.3442, 24.2677) ccw
  line L235 (-157.8442, 24.2677) -> (-157.8442, 10.2677)
  arc A232 (90.3928, 8.7677) -> (90.8928, 9.2677) centre (90.3928, 9.2677) ccw
  line L236 (90.3928, 8.7677) -> (77.3928, 8.7677)
  arc A233 (76.8928, 9.2677) -> (77.3928, 8.7677) centre (77.3928, 9.2677) ccw
  line L237 (76.8928, 9.2677) -> (76.8928, 22.2677)
  arc A234 (77.3928, 22.7677) -> (76.8928, 22.2677) centre (77.3928, 22.2677) ccw
  line L238 (77.3928, 22.7677) -> (90.3928, 22.7677)
  arc A235 (90.8928, 22.2677) -> (90.3928, 22.7677) centre (90.3928, 22.2677) ccw
  line L239 (90.8928, 22.2677) -> (90.8928, 9.2677)
  arc A236 (71.3428, -10.2823) -> (71.8428, -9.7823) centre (71.3428, -9.7823) ccw
  line L240 (71.3428, -10.2823) -> (58.3428, -10.2823)
  arc A237 (57.8428, -9.7823) -> (58.3428, -10.2823) centre (58.3428, -9.7823) ccw
  line L241 (57.8428, -9.7823) -> (57.8428, 3.2177)
  arc A238 (58.3428, 3.7177) -> (57.8428, 3.2177) centre (58.3428, 3.2177) ccw
  line L242 (58.3428, 3.7177) -> (71.3428, 3.7177)
  arc A239 (71.8428, 3.2177) -> (71.3428, 3.7177) centre (71.3428, 3.2177) ccw
  line L243 (71.8428, 3.2177) -> (71.8428, -9.7823)
  arc A240 (33.2428, -10.2823) -> (33.7428, -9.7823) centre (33.2428, -9.7823) ccw
  line L244 (33.2428, -10.2823) -> (20.2428, -10.2823)
  arc A241 (19.7428, -9.7823) -> (20.2428, -10.2823) centre (20.2428, -9.7823) ccw
  line L245 (19.7428, -9.7823) -> (19.7428, 3.2177)
  arc A242 (20.2428, 3.7177) -> (19.7428, 3.2177) centre (20.2428, 3.2177) ccw
  line L246 (20.2428, 3.7177) -> (33.2428, 3.7177)
  arc A243 (33.7428, 3.2177) -> (33.2428, 3.7177) centre (33.2428, 3.2177) ccw
  line L247 (33.7428, 3.2177) -> (33.7428, -9.7823)
  arc A244 (-4.8572, 8.7677) -> (-4.3572, 9.2677) centre (-4.8572, 9.2677) ccw
  line L248 (-4.8572, 8.7677) -> (-17.8572, 8.7677)
  arc A245 (-18.3572, 9.2677) -> (-17.8572, 8.7677) centre (-17.8572, 9.2677) ccw
  line L249 (-18.3572, 9.2677) -> (-18.3572, 22.2677)
  arc A246 (-17.8572, 22.7677) -> (-18.3572, 22.2677) centre (-17.8572, 22.2677) ccw
  line L250 (-17.8572, 22.7677) -> (-4.8572, 22.7677)
  arc A247 (-4.3572, 22.2677) -> (-4.8572, 22.7677) centre (-4.8572, 22.2677) ccw
  line L251 (-4.3572, 22.2677) -> (-4.3572, 9.2677)
  arc A248 (9.4303, 65.9177) -> (9.9303, 66.4177) centre (9.4303, 66.4177) ccw
  line L252 (9.4303, 65.9177) -> (-3.5697, 65.9177)
  arc A249 (-4.0697, 66.4177) -> (-3.5697, 65.9177) centre (-3.5697, 66.4177) ccw
  line L253 (-4.0697, 66.4177) -> (-4.0697, 79.4177)
  arc A250 (-3.5697, 79.9177) -> (-4.0697, 79.4177) centre (-3.5697, 79.4177) ccw
  line L254 (-3.5697, 79.9177) -> (9.4303, 79.9177)
  arc A251 (9.9303, 79.4177) -> (9.4303, 79.9177) centre (9.4303, 79.4177) ccw
  line L255 (9.9303, 79.4177) -> (9.9303, 66.4177)
  arc A252 (23.7178, 27.8177) -> (24.2178, 28.3177) centre (23.7178, 28.3177) ccw
  line L256 (23.7178, 27.8177) -> (10.7178, 27.8177)
  arc A253 (10.2178, 28.3177) -> (10.7178, 27.8177) centre (10.7178, 28.3177) ccw
  line L257 (10.2178, 28.3177) -> (10.2178, 41.3177)
  arc A254 (10.7178, 41.8177) -> (10.2178, 41.3177) centre (10.7178, 41.3177) ccw
  line L258 (10.7178, 41.8177) -> (23.7178, 41.8177)
  arc A255 (24.2178, 41.3177) -> (23.7178, 41.8177) centre (23.7178, 41.3177) ccw
  line L259 (24.2178, 41.3177) -> (24.2178, 28.3177)
  arc A256 (-62.0072, -10.2823) -> (-61.5072, -9.7823) centre (-62.0072, -9.7823) ccw
  line L260 (-62.0072, -10.2823) -> (-75.0072, -10.2823)
  arc A257 (-75.5072, -9.7823) -> (-75.0072, -10.2823) centre (-75.0072, -9.7823) ccw
  line L261 (-75.5072, -9.7823) -> (-75.5072, 3.2177)
  arc A258 (-75.0072, 3.7177) -> (-75.5072, 3.2177) centre (-75.0072, 3.2177) ccw
  line L262 (-75.0072, 3.7177) -> (-62.0072, 3.7177)
  arc A259 (-61.5072, 3.2177) -> (-62.0072, 3.7177) centre (-62.0072, 3.2177) ccw
  line L263 (-61.5072, 3.2177) -> (-61.5072, -9.7823)
  arc A260 (-62.0072, 8.7677) -> (-61.5072, 9.2677) centre (-62.0072, 9.2677) ccw
  line L264 (-62.0072, 8.7677) -> (-75.0072, 8.7677)
  arc A261 (-75.5072, 9.2677) -> (-75.0072, 8.7677) centre (-75.0072, 9.2677) ccw
  line L265 (-75.5072, 9.2677) -> (-75.5072, 22.2677)
  arc A262 (-75.0072, 22.7677) -> (-75.5072, 22.2677) centre (-75.0072, 22.2677) ccw
  line L266 (-75.0072, 22.7677) -> (-62.0072, 22.7677)
  arc A263 (-61.5072, 22.2677) -> (-62.0072, 22.7677) centre (-62.0072, 22.2677) ccw
  line L267 (-61.5072, 22.2677) -> (-61.5072, 9.2677)
  arc A264 (71.3428, 8.7677) -> (71.8428, 9.2677) centre (71.3428, 9.2677) ccw
  line L268 (71.3428, 8.7677) -> (58.3428, 8.7677)
  arc A265 (57.8428, 9.2677) -> (58.3428, 8.7677) centre (58.3428, 9.2677) ccw
  line L269 (57.8428, 9.2677) -> (57.8428, 22.2677)
  arc A266 (58.3428, 22.7677) -> (57.8428, 22.2677) centre (58.3428, 22.2677) ccw
  line L270 (58.3428, 22.7677) -> (71.3428, 22.7677)
  arc A267 (71.8428, 22.2677) -> (71.3428, 22.7677) centre (71.3428, 22.2677) ccw
  line L271 (71.8428, 22.2677) -> (71.8428, 9.2677)
  arc A268 (-147.7322, 27.8177) -> (-147.2322, 28.3177) centre (-147.7322, 28.3177) ccw
  line L272 (-147.7322, 27.8177) -> (-160.7322, 27.8177)
  arc A269 (-161.2322, 28.3177) -> (-160.7322, 27.8177) centre (-160.7322, 28.3177) ccw
  line L273 (-161.2322, 28.3177) -> (-161.2322, 41.3177)
  arc A270 (-160.7322, 41.8177) -> (-161.2322, 41.3177) centre (-160.7322, 41.3177) ccw
  line L274 (-160.7322, 41.8177) -> (-147.7322, 41.8177)
  arc A271 (-147.2322, 41.3177) -> (-147.7322, 41.8177) centre (-147.7322, 41.3177) ccw
  line L275 (-147.2322, 41.3177) -> (-147.2322, 28.3177)
  arc A272 (-150.1134, 65.9177) -> (-149.6134, 66.4177) centre (-150.1134, 66.4177) ccw
  line L276 (-150.1134, 65.9177) -> (-163.1134, 65.9177)
  arc A273 (-163.6134, 66.4177) -> (-163.1134, 65.9177) centre (-163.1134, 66.4177) ccw
  line L277 (-163.6134, 66.4177) -> (-163.6134, 79.4177)
  arc A274 (-163.1134, 79.9177) -> (-163.6134, 79.4177) centre (-163.1134, 79.4177) ccw
  line L278 (-163.1134, 79.9177) -> (-150.1134, 79.9177)
  arc A275 (-149.6134, 79.4177) -> (-150.1134, 79.9177) centre (-150.1134, 79.4177) ccw
  line L279 (-149.6134, 79.4177) -> (-149.6134, 66.4177)
  arc A276 (-179.8389, 47.8677) -> (-179.3389, 48.3677) centre (-179.8389, 48.3677) ccw
  line L280 (-179.8389, 47.8677) -> (-185.8389, 47.8677)
  arc A277 (-186.3389, 48.3677) -> (-185.8389, 47.8677) centre (-185.8389, 48.3677) ccw
  line L281 (-186.3389, 48.3677) -> (-186.3389, 62.3677)
  arc A278 (-185.8389, 62.8677) -> (-186.3389, 62.3677) centre (-185.8389, 62.3677) ccw
  line L282 (-185.8389, 62.8677) -> (-179.8389, 62.8677)
  arc A279 (-179.3389, 62.3677) -> (-179.8389, 62.8677) centre (-179.8389, 62.3677) ccw
  line L283 (-179.3389, 62.3677) -> (-179.3389, 48.3677)
  arc A280 (38.0053, 46.8677) -> (38.5053, 47.3677) centre (38.0053, 47.3677) ccw
  line L284 (38.0053, 46.8677) -> (25.0053, 46.8677)
  arc A281 (24.5053, 47.3677) -> (25.0053, 46.8677) centre (25.0053, 47.3677) ccw
  line L285 (24.5053, 47.3677) -> (24.5053, 60.3677)
  arc A282 (25.0053, 60.8677) -> (24.5053, 60.3677) centre (25.0053, 60.3677) ccw
  line L286 (25.0053, 60.8677) -> (38.0053, 60.8677)
  arc A283 (38.5053, 60.3677) -> (38.0053, 60.8677) centre (38.0053, 60.3677) ccw
  line L287 (38.5053, 60.3677) -> (38.5053, 47.3677)
  arc A284 (-90.5822, 27.8177) -> (-90.0822, 28.3177) centre (-90.5822, 28.3177) ccw
  line L288 (-90.5822, 27.8177) -> (-103.5822, 27.8177)
  arc A285 (-104.0822, 28.3177) -> (-103.5822, 27.8177) centre (-103.5822, 28.3177) ccw
  line L289 (-104.0822, 28.3177) -> (-104.0822, 41.3177)
  arc A286 (-103.5822, 41.8177) -> (-104.0822, 41.3177) centre (-103.5822, 41.3177) ccw
  line L290 (-103.5822, 41.8177) -> (-90.5822, 41.8177)
  arc A287 (-90.0822, 41.3177) -> (-90.5822, 41.8177) centre (-90.5822, 41.3177) ccw
  line L291 (-90.0822, 41.3177) -> (-90.0822, 28.3177)
  arc A288 (47.5303, 65.9177) -> (48.0303, 66.4177) centre (47.5303, 66.4177) ccw
  line L292 (47.5303, 65.9177) -> (34.5303, 65.9177)
  arc A289 (34.0303, 66.4177) -> (34.5303, 65.9177) centre (34.5303, 66.4177) ccw
  line L293 (34.0303, 66.4177) -> (34.0303, 79.4177)
  arc A290 (34.5303, 79.9177) -> (34.0303, 79.4177) centre (34.5303, 79.4177) ccw
  line L294 (34.5303, 79.9177) -> (47.5303, 79.9177)
  arc A291 (48.0303, 79.4177) -> (47.5303, 79.9177) centre (47.5303, 79.4177) ccw
  line L295 (48.0303, 79.4177) -> (48.0303, 66.4177)
  arc A292 (57.0553, 46.8677) -> (57.5553, 47.3677) centre (57.0553, 47.3677) ccw
  line L296 (57.0553, 46.8677) -> (44.0553, 46.8677)
  arc A293 (43.5553, 47.3677) -> (44.0553, 46.8677) centre (44.0553, 47.3677) ccw
  line L297 (43.5553, 47.3677) -> (43.5553, 60.3677)
  arc A294 (44.0553, 60.8677) -> (43.5553, 60.3677) centre (44.0553, 60.3677) ccw
  line L298 (44.0553, 60.8677) -> (57.0553, 60.8677)
  arc A295 (57.5553, 60.3677) -> (57.0553, 60.8677) centre (57.0553, 60.3677) ccw
  line L299 (57.5553, 60.3677) -> (57.5553, 47.3677)
  arc A296 (-81.0572, 8.7677) -> (-80.5572, 9.2677) centre (-81.0572, 9.2677) ccw
  line L300 (-81.0572, 8.7677) -> (-94.0572, 8.7677)
  arc A297 (-94.5572, 9.2677) -> (-94.0572, 8.7677) centre (-94.0572, 9.2677) ccw
  line L301 (-94.5572, 9.2677) -> (-94.5572, 22.2677)
  arc A298 (-94.0572, 22.7677) -> (-94.5572, 22.2677) centre (-94.0572, 22.2677) ccw
  line L302 (-94.0572, 22.7677) -> (-81.0572, 22.7677)
  arc A299 (-80.5572, 22.2677) -> (-81.0572, 22.7677) centre (-81.0572, 22.2677) ccw
  line L303 (-80.5572, 22.2677) -> (-80.5572, 9.2677)
  arc A300 (28.4803, 65.9177) -> (28.9803, 66.4177) centre (28.4803, 66.4177) ccw
  line L304 (28.4803, 65.9177) -> (15.4803, 65.9177)
  arc A301 (14.9803, 66.4177) -> (15.4803, 65.9177) centre (15.4803, 66.4177) ccw
  line L305 (14.9803, 66.4177) -> (14.9803, 79.4177)
  arc A302 (15.4803, 79.9177) -> (14.9803, 79.4177) centre (15.4803, 79.4177) ccw
  line L306 (15.4803, 79.9177) -> (28.4803, 79.9177)
  arc A303 (28.9803, 79.4177) -> (28.4803, 79.9177) centre (28.4803, 79.4177) ccw
  line L307 (28.9803, 79.4177) -> (28.9803, 66.4177)
  arc A304 (61.8178, 27.8177) -> (62.3178, 28.3177) centre (61.8178, 28.3177) ccw
  line L308 (61.8178, 27.8177) -> (48.8178, 27.8177)
  arc A305 (48.3178, 28.3177) -> (48.8178, 27.8177) centre (48.8178, 28.3177) ccw
  line L309 (48.3178, 28.3177) -> (48.3178, 41.3177)
  arc A306 (48.8178, 41.8177) -> (48.3178, 41.3177) centre (48.8178, 41.3177) ccw
  line L310 (48.8178, 41.8177) -> (61.8178, 41.8177)
  arc A307 (62.3178, 41.3177) -> (61.8178, 41.8177) centre (61.8178, 41.3177) ccw
  line L311 (62.3178, 41.3177) -> (62.3178, 28.3177)
  arc A308 (-123.9197, 65.9177) -> (-123.4197, 66.4177) centre (-123.9197, 66.4177) ccw
  line L312 (-123.9197, 65.9177) -> (-136.9197, 65.9177)
  arc A309 (-137.4197, 66.4177) -> (-136.9197, 65.9177) centre (-136.9197, 66.4177) ccw
  line L313 (-137.4197, 66.4177) -> (-137.4197, 79.4177)
  arc A310 (-136.9197, 79.9177) -> (-137.4197, 79.4177) centre (-136.9197, 79.4177) ccw
  line L314 (-136.9197, 79.9177) -> (-123.9197, 79.9177)
  arc A311 (-123.4197, 79.4177) -> (-123.9197, 79.9177) centre (-123.9197, 79.4177) ccw
  line L315 (-123.4197, 79.4177) -> (-123.4197, 66.4177)
  arc A312 (-19.1447, 46.8677) -> (-18.6447, 47.3677) centre (-19.1447, 47.3677) ccw
  line L316 (-19.1447, 46.8677) -> (-32.1447, 46.8677)
  arc A313 (-32.6447, 47.3677) -> (-32.1447, 46.8677) centre (-32.1447, 47.3677) ccw
  line L317 (-32.6447, 47.3677) -> (-32.6447, 60.3677)
  arc A314 (-32.1447, 60.8677) -> (-32.6447, 60.3677) centre (-32.1447, 60.3677) ccw
  line L318 (-32.1447, 60.8677) -> (-19.1447, 60.8677)
  arc A315 (-18.6447, 60.3677) -> (-19.1447, 60.8677) centre (-19.1447, 60.3677) ccw
  line L319 (-18.6447, 60.3677) -> (-18.6447, 47.3677)
  arc A316 (-195.3572, -10.2823) -> (-194.8572, -9.7823) centre (-195.3572, -9.7823) ccw
  line L320 (-195.3572, -10.2823) -> (-208.3572, -10.2823)
  arc A317 (-208.8572, -9.7823) -> (-208.3572, -10.2823) centre (-208.3572, -9.7823) ccw
  line L321 (-208.8572, -9.7823) -> (-208.8572, 3.2177)
  arc A318 (-208.3572, 3.7177) -> (-208.8572, 3.2177) centre (-208.3572, 3.2177) ccw
  line L322 (-208.3572, 3.7177) -> (-195.3572, 3.7177)
  arc A319 (-194.8572, 3.2177) -> (-195.3572, 3.7177) centre (-195.3572, 3.2177) ccw
  line L323 (-194.8572, 3.2177) -> (-194.8572, -9.7823)
  arc A320 (-52.4822, 27.8177) -> (-51.9822, 28.3177) centre (-52.4822, 28.3177) ccw
  line L324 (-52.4822, 27.8177) -> (-65.4822, 27.8177)
  arc A321 (-65.9822, 28.3177) -> (-65.4822, 27.8177) centre (-65.4822, 28.3177) ccw
  line L325 (-65.9822, 28.3177) -> (-65.9822, 41.3177)
  arc A322 (-65.4822, 41.8177) -> (-65.9822, 41.3177) centre (-65.4822, 41.3177) ccw
  line L326 (-65.4822, 41.8177) -> (-52.4822, 41.8177)
  arc A323 (-51.9822, 41.3177) -> (-52.4822, 41.8177) centre (-52.4822, 41.3177) ccw
  line L327 (-51.9822, 41.3177) -> (-51.9822, 28.3177)
  arc A324 (-195.3572, 65.9177) -> (-194.8572, 66.4177) centre (-195.3572, 66.4177) ccw
  line L328 (-195.3572, 65.9177) -> (-208.3572, 65.9177)
  arc A325 (-208.8572, 66.4177) -> (-208.3572, 65.9177) centre (-208.3572, 66.4177) ccw
  line L329 (-208.8572, 66.4177) -> (-208.8572, 79.4177)
  arc A326 (-208.3572, 79.9177) -> (-208.8572, 79.4177) centre (-208.3572, 79.4177) ccw
  line L330 (-208.3572, 79.9177) -> (-195.3572, 79.9177)
  arc A327 (-194.8572, 79.4177) -> (-195.3572, 79.9177) centre (-195.3572, 79.4177) ccw
  line L331 (-194.8572, 79.4177) -> (-194.8572, 66.4177)
  arc A328 (-31.0509, 84.9677) -> (-30.5509, 85.4677) centre (-31.0509, 85.4677) ccw
  line L332 (-31.0509, 84.9677) -> (-44.0509, 84.9677)
  arc A329 (-44.5509, 85.4677) -> (-44.0509, 84.9677) centre (-44.0509, 85.4677) ccw
  line L333 (-44.5509, 85.4677) -> (-44.5509, 98.4677)
  arc A330 (-44.0509, 98.9677) -> (-44.5509, 98.4677) centre (-44.0509, 98.4677) ccw
  line L334 (-44.0509, 98.9677) -> (-31.0509, 98.9677)
  arc A331 (-30.5509, 98.4677) -> (-31.0509, 98.9677) centre (-31.0509, 98.4677) ccw
  line L335 (-30.5509, 98.4677) -> (-30.5509, 85.4677)
  arc A332 (14.1928, -10.2823) -> (14.6928, -9.7823) centre (14.1928, -9.7823) ccw
  line L336 (14.1928, -10.2823) -> (1.1928, -10.2823)
  arc A333 (0.6928, -9.7823) -> (1.1928, -10.2823) centre (1.1928, -9.7823) ccw
  line L337 (0.6928, -9.7823) -> (0.6928, 3.2177)
  arc A334 (1.1928, 3.7177) -> (0.6928, 3.2177) centre (1.1928, 3.2177) ccw
  line L338 (1.1928, 3.7177) -> (14.1928, 3.7177)
  arc A335 (14.6928, 3.2177) -> (14.1928, 3.7177) centre (14.1928, 3.2177) ccw
  line L339 (14.6928, 3.2177) -> (14.6928, -9.7823)
  arc A336 (-95.3447, 46.8677) -> (-94.8447, 47.3677) centre (-95.3447, 47.3677) ccw
  line L340 (-95.3447, 46.8677) -> (-108.3447, 46.8677)